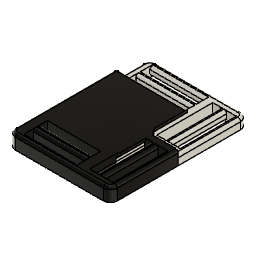
Bickle v11 (Autodesk Fusion 360 design; units mm, degrees)
Autodesk Fusion 360 part; units mm, degrees
sketch "Sketch1" plane through (0, 0, 0) normal (0, 0, 1) x (1, 0, 0)
  line L0 (0, 0) -> (50.5, 0)
  line L1 (0, 0) -> (5, 0)
  line L2 (5, 0) -> (5, -5) construction
  line L3 (0, 0) -> (0, -5)
  line L4 (50.5, 0) -> (50.5, -5)
  line L5 (50.5, -5) -> (45.5, -5)
  line L6 (45.5, -5) -> (45.5, 0) construction
  line L7 (45.5, -5) -> (0, -5)
  line L8 (0, -5) -> (0, -10)
  line L9 (0, -10) -> (50.5, -10)
  line L10 (50.5, -5) -> (50.5, -10)
  line L11 (0, 0) -> (0, 5)
  line L12 (0, 5) -> (51, 5)
  line L13 (50.5, 0) -> (50.5, 5)
  line L14 (0, -10) -> (0, -65)
  line L15 (50.5, -10) -> (50.5, -65)
  line L16 (50.5, -65) -> (0, -65)
  line L17 (45.5, 5) -> (45.5, -10)
  line L18 (5, -5) -> (5, -10)
  line L19 (5, 0) -> (5, 5)
  line L20 (50.5, 5) -> (50.5, 10)
  line L21 (50.5, 10) -> (0, 10)
  line L22 (0, 10) -> (0, 5)
  dimension "d1" = 50.5
  dimension "d2" = 5
  dimension "d3" = 5
  dimension "d4" = 5
  dimension "d5" = 5
  dimension "d6" = 5
  dimension "d7" = 5
  dimension "d8" = 5
  dimension "d11" = 55
  dimension "d12" = 55
  dimension "d13" = 5
  constraint coincident L0.start L1.start
  constraint horizontal L0
  constraint parallel L0 L1
  constraint perpendicular L0 L2
  constraint perpendicular L1 L3
  constraint perpendicular L0 L4
  constraint perpendicular L4 L5
  constraint coincident L0 L6.end
  constraint perpendicular L0 L6
  constraint perpendicular L7 L8
  constraint perpendicular L8 L9
  constraint coincident L9 L10.end
  constraint perpendicular L9 L10
  constraint perpendicular L1 L11
  constraint perpendicular L11 L12
  constraint coincident L12 L13.end
  constraint perpendicular L12 L13
  constraint perpendicular L9 L14
  constraint perpendicular L9 L15
  constraint coincident L12 L17.start
  constraint coincident L9 L17.end
  constraint perpendicular L9 L17
  constraint coincident L9 L18.end
  constraint perpendicular L9 L18
  constraint coincident L12 L19.end
  constraint perpendicular L12 L19
  constraint perpendicular L12 L20
  constraint perpendicular L20 L21
  constraint coincident L12 L11.end
  constraint perpendicular L12 L22
  measures "d1" distance of L0.start L0.end
  measures "d2" distance of L0.start L1.end
  measures "d3" distance of L1.end L2.end
  measures "d4" distance of L0.start L3.end
  measures "d5" distance of L0.end L4.end
  measures "d6" distance of L4.end L5.end
  measures "d7" distance of L3.end L8.end
  measures "d8" distance of L0.start L11.end
  measures "d11" distance of L8.end L14.end
  measures "d12" distance of L9.end L15.end
  measures "d13" distance of L13.end L20.end
extrude "Extrude2" add sketch "Sketch1" along normal blind 7 contours L0 L1 L11 L12 L19 | L0 L1 L3 L7 L17 | L7 L8 L9 L18 | L12 L20 L21 L22 | L0 L12 L13 L17 | L0 L4 L5 L17 | L9 L14 L15 L16 | L5 L9 L10 L17 makes body 1
fillet "Fillet1" radius 2 4 edges at (25.25, 0, 0) (25.25, -5, 0) (25.25, -5, 7) (25.25, 0, 7) on bodies 1
sketch "Sketch2" plane through (0, 0, 0) normal (0, 0, -1) x (1, 0, 0)
  line L0 (45.5, 10) -> (45.5, 3)
  line L1 (45.5, 3) -> (5, 3)
  line L2 (5, 3) -> (5, 10)
  line L3 (5, 10) -> (45.5, 10)
  line L4 (5, -5) -> (5, 2)
  line L5 (5, 2) -> (45.5, 2)
  line L6 (45.5, 2) -> (45.5, -5)
  line L7 (45.5, -5) -> (5, -5)
  line L8 (50.5, -10) -> (50.5, 65)
  line L9 (50.5, 65) -> (0, 65)
  line L10 (0, 65) -> (0, -10)
  line L11 (0, -10) -> (50.5, -10)
  line L12 (50.5, -10) -> (70.5, -10)
  line L13 (70.5, -10) -> (70.5, 40.5)
  line L14 (70.5, 40.5) -> (50.5, 65)
  line L15 (70.5, 40.5) -> (50.5, 40.5)
  line L16 (50.5, -10) -> (55.5, -10)
  line L17 (55.5, -10) -> (60.5, -10)
  line L18 (60.5, -10) -> (65.5, -10)
  line L19 (65.5, -10) -> (65.5, 40.5)
  line L20 (60.5, -10) -> (60.5, 40.5)
  line L21 (55.5, -10) -> (55.5, 40.5)
  line L22 (50.5, -10) -> (50.5, -5)
  line L23 (50.5, -5) -> (70.5, -5)
  line L24 (70.5, 40.5) -> (70.5, 35.5)
  line L25 (70.5, 35.5) -> (50.5, 35.5)
  dimension "d18" = 20
  dimension "d19" = 50.5
  dimension "d20" = 5
  dimension "d21" = 5
  dimension "d22" = 5
  dimension "d23" = 5
  constraint coincident L8.start L11.end
  constraint perpendicular L8 L12
  constraint perpendicular L12 L13
  constraint coincident L8.end L9.start
  constraint coincident L8 L15.end
  constraint perpendicular L8 L15
  constraint perpendicular L8 L16
  constraint parallel L12 L17
  constraint coincident L12 L18.end
  constraint coincident L15 L19.end
  constraint perpendicular L15 L19
  constraint midpoint L15 L20.end
  constraint coincident L15 L21.end
  constraint perpendicular L15 L21
  constraint coincident L8 L22.end
  constraint perpendicular L16 L22
  constraint coincident L13 L23.end
  constraint perpendicular L13 L23
  constraint perpendicular L15 L24
  constraint coincident L8 L25.end
  constraint perpendicular L8 L25
  measures "d18" distance of L8.start L12.end
  measures "d19" distance of L12.end L13.end
  measures "d20" distance of L8.start L16.end
  measures "d21" distance of L16.end L17.end
  measures "d22" distance of L17.end L18.end
  measures "d23" distance of L13.end L24.end
extrude "Extrude3" add sketch "Sketch2" against normal up to surface (7 mm away) contours L8 L12 L16 L21 L22 L23 | L12 L17 L20 L21 L23 | L8 L15 L21 L25 | L20 L21 L23 L25 | L12 L18 L19 L20 L23 | L15 L20 L21 L25 | L12 L13 L19 L23 | L15 L19 L20 L25 | L13 L19 L23 L25 | L13 L15 L19 L24 L25 bodies 1
fillet "Fillet2" radius 2 4 edges at (60.5, -15.25, 7) (60.5, -15.25, 0) (55.5, -15.25, 7) (55.5, -15.25, 0) on bodies 1
sketch "Sketch3" plane through (0, 0, 7) normal (0, 0, 1) x (-1, 0, 0)
  line L0 (-70.5, -10) -> (0, -10)
  line L1 (0, -10) -> (0, 65)
  line L2 (0, 65) -> (-50.5, 65)
  line L3 (-70.5, 40.5) -> (-70.5, -10)
  line L4 (-65.5, 35.5) -> (-58.5, 35.5)
  line L5 (-58.5, 35.5) -> (-58.5, -5)
  line L6 (-58.5, -5) -> (-65.5, -5)
  line L7 (-65.5, -5) -> (-65.5, 35.5)
  line L8 (-5, 2) -> (-5, -5)
  line L9 (-5, -5) -> (-45.5, -5)
  line L10 (-45.5, -5) -> (-45.5, 2)
  line L11 (-45.5, 2) -> (-5, 2)
  line L12 (-45.5, 3) -> (-45.5, 10)
  line L13 (-45.5, 10) -> (-5, 10)
  line L14 (-5, 10) -> (-5, 3)
  line L15 (-5, 3) -> (-45.5, 3)
  line L16 (-50.5, -5) -> (-57.5, -5)
  line L17 (-57.5, -5) -> (-57.5, 35.5)
  line L18 (-57.5, 35.5) -> (-50.5, 35.5)
  line L19 (-50.5, 65) -> (-50.5, 40.5)
  line L20 (-25.25, 10) -> (-25.25, 65) construction
  line L21 (-45.5, 10) -> (-51, 10) construction
  line L22 (-50.5, 65) -> (-50.5, 10) construction
  circle A0 centre (-25.25, 37.5) radius 12.25
  line L23 (-70.5, 40.5) -> (0, 40.5) construction
  line L24 (-25.25, 49.75) -> (-25.25, 47.75) construction
  line L25 (-25.25, 47.75) -> (-18.5418, 47.75)
  line L26 (-25.25, 37.5) -> (-13, 37.5) construction
  line L27 (-18.5418, 47.75) -> (-13, 37.5)
  line L28 (-25.25, 37.5) -> (-39, 37.5) construction
  line L29 (-25.25, 47.75) -> (-31.9582, 47.75)
  line L30 (-31.9582, 47.75) -> (-37.5, 37.5)
  line L31 (-21.8959, 47.75) -> (-21.8959, 65)
  line L32 (-28.6041, 47.75) -> (-28.6041, 65)
  line L33 (-21.8959, 47.75) -> (-21.8959, 52.75)
  line L34 (-21.8959, 52.75) -> (-28.6041, 52.75)
  line L35 (-50.5, 40.5) -> (-70.5, 40.5)
  line L36 (-50.5, 35.5) -> (-50.5, -5)
  dimension "d28" = 2
  dimension "d31" = 5
  dimension "d38" = 24.5
  constraint midpoint L13 L20.start
  constraint midpoint L2 L20.end
  constraint coincident L12.end L13.start
  constraint perpendicular L19 L21
  constraint coincident L2.end L19.start
  constraint coincident L21 L22.end
  constraint coincident L19 L22.end
  constraint midpoint L20 A0.centre
  constraint coincident L3.start L23.start
  constraint coincident L1 L23.end
  constraint perpendicular L1 L23
  constraint coincident A0 L24.start
  constraint coincident L20 L24.start
  constraint parallel L20 L24
  constraint coincident A0 L25.end
  constraint perpendicular L24 L25
  constraint coincident A0.centre L26.start
  constraint coincident A0 L26.end
  constraint perpendicular L20 L26
  constraint perpendicular L20 L28
  constraint perpendicular L24 L29
  constraint coincident A0 L29.end
  constraint coincident L29 L30.start
  constraint coincident A0 L30.end
  constraint coincident L28 L30.end
  constraint midpoint L25 L31.start
  constraint coincident L2 L31.end
  constraint perpendicular L2 L31
  constraint midpoint L29 L32.start
  constraint coincident L2 L32.end
  constraint perpendicular L2 L32
  constraint perpendicular L25 L33
  constraint coincident L32 L34.end
  constraint perpendicular L32 L34
  measures "d28" distance of L24.start L24.end
  measures "d31" distance of L31.start L33.end
  measures "d38" diameter of A0
extrude "Extrude4" cut sketch "Sketch3" against normal blind 5 contours A0 L31 L32 L33 L34 | A0 L25 L29 L31 L32 L33 | A0 L25 L27 L29 L30 bodies 1
sketch "Sketch4" plane through (0, 0, 2) normal (0, 0, 1) x (-1, 0, 0)
  line L0 (-21.8959, 47.75) -> (-21.8959, 52.75)
  line L1 (-21.8959, 52.75) -> (-28.6041, 52.75)
  line L2 (-28.6041, 52.75) -> (-28.6041, 47.75)
  line L3 (-28.6041, 47.75) -> (-31.9582, 47.75)
  line L4 (-31.9582, 47.75) -> (-37.5, 37.5)
  arc A0 (-37.5, 37.5) -> (-13, 37.5) centre (-25.25, 37.5) ccw
  line L5 (-13, 37.5) -> (-18.5418, 47.75)
  line L6 (-18.5418, 47.75) -> (-21.8959, 47.75)
  circle A1 centre (-25.25, 37.5) radius 12.25
  line L7 (-25.25, 37.5) -> (-25.25, 52.75)
  line L8 (-25.25, 37.5) -> (-25.25, 47.5)
  circle A2 centre (-25.25, 47.5) radius 12.25
  line L9 (-13, 37.5) -> (-13, 47.5)
  line L10 (-37.5, 37.5) -> (-37.5, 47.5)
  dimension "d32" = 10
  dimension "d33" = 24.5
  dimension "d34" = 24.5
  constraint concentric A0 A1
  constraint coincident A0.centre A1.centre
  constraint midpoint L1 L7.end
  constraint parallel L7 L8
  constraint coincident L8.end A2.centre
  constraint coincident A0.end L5.start
  constraint coincident A2 L9.end
  constraint tangent A2 L9
  constraint coincident L4.end A0.start
  constraint coincident A2 L10.end
  constraint tangent A2 L10
  measures "d32" distance of A0.centre L8.end
  measures "d33" diameter of A1
  measures "d34" diameter of A2
extrude "Extrude5" cut sketch "Sketch4" along normal blind 3 contours L0 L2 L3 L4 L5 L6 A1 A2 | L0 L6 A1 | L0 L1 A1 L7 | L0 L1 L2 A1 A2 | L5 A1 A2 | L1 L2 A1 L7 | L5 A1 A2 | A1 A2 L9 | L2 L3 A1 | L4 A1 A2 | L4 A1 A2 | A1 A2 L10 bodies 1
sketch "Sketch1 (2)" plane through (0, 0, 2) normal (0, 0, 1) x (-1, 0, 0) in component "Topo"
  arc A0 (-37.5, 37.5) -> (-13, 37.5) centre (-25.25, 37.5) ccw
  line L0 (-13, 37.5) -> (-13, 47.5)
  arc A1 (-13, 47.5) -> (-37.5, 47.5) centre (-25.25, 47.5) ccw
  line L1 (-37.5, 47.5) -> (-37.5, 37.5)
  circle A2 centre (-25.25, 37.5) radius 10.7848
  point P0 (-28.6041, 47.75)
  constraint concentric A0 A2
  constraint coincident P0 A2
extrude "Extrude1" add sketch "Sketch1 (2)" along normal blind 2 separate body contours A2 makes body 2 in component "Topo"
fillet "Fillet3" radius 1 2 edges at (21.8959, -47.75, 6) (28.6041, -47.75, 6) on bodies 1
sketch "Sketch2 (2)" plane through (0, 0, 4) normal (0, 0, 1) x (-1, 0, 0) in component "Topo"
  circle A0 centre (-25.25, 37.5) radius 10.7848
  line L0 (-28.6041, 41.75) -> (-21.8959, 41.75)
  line L1 (-21.8959, 41.75) -> (-21.8959, 37.75)
  line L2 (-20.8959, 36.75) -> (-18.5418, 36.75)
  line L3 (-18.5418, 36.75) -> (-13, 26.5)
  arc A1 (-37.5, 26.5) -> (-13, 26.5) centre (-25.25, 26.5) ccw
  line L4 (-37.5, 26.5) -> (-31.9582, 36.75)
  line L5 (-31.9582, 36.75) -> (-29.6041, 36.75)
  line L6 (-28.6041, 37.75) -> (-28.6041, 41.75)
  line L7 (-70.5, -21) -> (0, -21)
  line L8 (0, -21) -> (0, 54)
  line L9 (0, 54) -> (-50.5, 54)
  line L10 (-70.5, 29.5) -> (-70.5, -21)
  line L11 (-65.5, 24.5) -> (-58.5, 24.5)
  line L12 (-58.5, 24.5) -> (-58.5, -16)
  line L13 (-58.5, -16) -> (-65.5, -16)
  line L14 (-65.5, -16) -> (-65.5, 24.5)
  line L15 (-5, -9) -> (-5, -16)
  line L16 (-5, -16) -> (-45.5, -16)
  line L17 (-45.5, -16) -> (-45.5, -9)
  line L18 (-45.5, -9) -> (-5, -9)
  line L19 (-45.5, -8) -> (-45.5, -1)
  line L20 (-45.5, -1) -> (-5, -1)
  line L21 (-5, -1) -> (-5, -8)
  line L22 (-5, -8) -> (-45.5, -8)
  line L23 (-50.5, -16) -> (-57.5, -16)
  line L24 (-57.5, -16) -> (-57.5, 24.5)
  line L25 (-57.5, 24.5) -> (-50.5, 24.5)
  line L26 (-50.5, 54) -> (-50.5, 29.5)
  arc A2 (-29.6041, 36.75) -> (-28.6041, 37.75) centre (-29.6041, 37.75) ccw
  arc A3 (-21.8959, 37.75) -> (-20.8959, 36.75) centre (-20.8959, 37.75) ccw
  line L27 (-22.3959, 41.25) -> (-22.3959, 37.75)
  arc A4 (-22.3959, 37.75) -> (-20.8959, 36.25) centre (-20.8959, 37.75) ccw
  line L28 (-20.8959, 36.25) -> (-18.8399, 36.25)
  line L29 (-18.8399, 36.25) -> (-13.5007, 26.3747)
  arc A5 (-36.9993, 26.3747) -> (-13.5007, 26.3747) centre (-25.25, 26.5) ccw
  line L30 (-36.9993, 26.3747) -> (-31.6601, 36.25)
  line L31 (-31.6601, 36.25) -> (-29.6041, 36.25)
  arc A6 (-29.6041, 36.25) -> (-28.1041, 37.75) centre (-29.6041, 37.75) ccw
  line L32 (-28.1041, 37.75) -> (-28.1041, 41.25)
  line L33 (-28.1041, 41.25) -> (-22.3959, 41.25)
  line L34 (-50.5, 29.5) -> (-70.5, 29.5)
  line L35 (-50.5, 24.5) -> (-50.5, -16)
  dimension "d43" = 0.5
extrude "Extrude2'" add sketch "Sketch2 (2)" along normal up to surface (3 mm away) contours A0 L27 A4 L28 L29 L30 L31 A6 L32 L33 bodies 2 in component "Topo"
extrude "Extrude3'" add 1 faces at (25.25, -33.316, 7) along direction (0, 0, 1) blind 1 on bodies 2 bodies 2 in component "Topo"
move_body "Move1" bodies 2 to x (1, 0, 0) y (0, 1, 0) z (0, 0, 1) at (0, 11, 0) in component "Topo"
sketch "Sketch4 (2)" plane through (0, 0, 8) normal (0, 0, 1) x (-1, 0, 0) in component "Topo"
  line L0 (-31.6601, 25.25) -> (-34.2209, 20.5137)
  arc A0 (-34.2209, 20.5137) -> (-16.2791, 20.5137) centre (-25.25, 26.5) ccw
  line L1 (-16.2791, 20.5137) -> (-18.8399, 25.25)
  line L2 (-18.8399, 25.25) -> (-20.8959, 25.25)
  arc A1 (-22.3959, 26.75) -> (-20.8959, 25.25) centre (-20.8959, 26.75) ccw
  line L3 (-22.3959, 26.75) -> (-22.3959, 30.25)
  line L4 (-22.3959, 30.25) -> (-28.1041, 30.25)
  line L5 (-28.1041, 30.25) -> (-28.1041, 26.75)
  arc A2 (-29.6041, 25.25) -> (-28.1041, 26.75) centre (-29.6041, 26.75) ccw
  line L6 (-29.6041, 25.25) -> (-31.6601, 25.25)
  arc A3 (-29.6041, 36.75) -> (-28.6041, 37.75) centre (-29.6041, 37.75) ccw
  line L7 (-28.6041, 37.75) -> (-28.6041, 41.75)
  line L8 (-28.6041, 41.75) -> (-21.8959, 41.75)
  line L9 (-21.8959, 41.75) -> (-21.8959, 37.75)
  arc A4 (-21.8959, 37.75) -> (-20.8959, 36.75) centre (-20.8959, 37.75) ccw
  line L10 (-20.8959, 36.75) -> (-18.5418, 36.75)
  line L11 (-18.5418, 36.75) -> (-13, 26.5)
  arc A5 (-37.5, 26.5) -> (-13, 26.5) centre (-25.25, 26.5) ccw
  line L12 (-37.5, 26.5) -> (-31.9582, 36.75)
  line L13 (-31.9582, 36.75) -> (-29.6041, 36.75)
  line L14 (-70.5, -21) -> (0, -21)
  line L15 (0, -21) -> (0, 54)
  line L16 (0, 54) -> (-50.5, 54)
  line L17 (-70.5, 29.5) -> (-70.5, -21)
  line L18 (-65.5, 24.5) -> (-58.5, 24.5)
  line L19 (-58.5, 24.5) -> (-58.5, -16)
  line L20 (-58.5, -16) -> (-65.5, -16)
  line L21 (-65.5, -16) -> (-65.5, 24.5)
  line L22 (-5, -9) -> (-5, -16)
  line L23 (-5, -16) -> (-45.5, -16)
  line L24 (-45.5, -16) -> (-45.5, -9)
  line L25 (-45.5, -9) -> (-5, -9)
  line L26 (-45.5, -8) -> (-45.5, -1)
  line L27 (-45.5, -1) -> (-5, -1)
  line L28 (-5, -1) -> (-5, -8)
  line L29 (-5, -8) -> (-45.5, -8)
  line L30 (-50.5, -16) -> (-57.5, -16)
  line L31 (-57.5, -16) -> (-57.5, 24.5)
  line L32 (-57.5, 24.5) -> (-50.5, 24.5)
  line L33 (-50.5, 54) -> (-50.5, 29.5)
  line L34 (0, -1) -> (0, 1)
  line L35 (-50.5, 24.5) -> (-48.5, 24.5)
  line L36 (-48.5, 24.5) -> (-48.5, 54)
  line L37 (-48.5, 24.5) -> (-48.5, -2)
  line L38 (0, 1) -> (-48.5, 1)
  line L39 (-48.5, 54) -> (-48.5, 59)
  line L40 (0, 54) -> (0, 59)
  line L41 (0, 59) -> (-48.5, 59)
  line L42 (0, 59) -> (0, 64)
  line L43 (0, 64) -> (0, 69)
  line L44 (0, 69) -> (0, 74)
  line L45 (0, 64) -> (-49, 64)
  line L46 (0, 69) -> (-51, 69)
  line L47 (0, 74) -> (-52, 74)
  line L48 (-48.5, 59) -> (-48.5, 74)
  line L49 (0, 54) -> (-5, 54)
  line L50 (-5, 54) -> (-5, 74)
  line L51 (-48.5, 54) -> (-43.5, 54)
  line L52 (-43.5, 54) -> (-43.5, 74)
  line L53 (-70.5, 29.5) -> (-48.5, 29.5)
  line L54 (-50.5, 29.5) -> (-70.5, 29.5)
  line L55 (-50.5, 24.5) -> (-50.5, -16)
  line L56 (-31.6601, 25.25) -> (-34.2209, 20.5137)
  arc A6 (-34.2209, 20.5137) -> (-16.2791, 20.5137) centre (-25.25, 26.5) ccw
  line L57 (-16.2791, 20.5137) -> (-18.8399, 25.25)
  line L58 (-18.8399, 25.25) -> (-20.8959, 25.25)
  arc A7 (-22.3959, 26.75) -> (-20.8959, 25.25) centre (-20.8959, 26.75) ccw
  line L59 (-22.3959, 26.75) -> (-22.3959, 30.25)
  line L60 (-22.3959, 30.25) -> (-28.1041, 30.25)
  line L61 (-28.1041, 30.25) -> (-28.1041, 26.75)
  arc A8 (-29.6041, 25.25) -> (-28.1041, 26.75) centre (-29.6041, 26.75) ccw
  line L62 (-29.6041, 25.25) -> (-31.6601, 25.25)
  line L63 (0, 79) -> (-53, 79)
  line L64 (-48.5, 74) -> (-48.5, 79)
  line L65 (0, 79) -> (0, 74)
  line L66 (-43.5, 74) -> (-43.5, 79)
  line L67 (-5, 74) -> (-5, 79)
  dimension "d48" = 2
  dimension "d49" = 2
  dimension "d52" = 5
  dimension "d53" = 5
  dimension "d54" = 5
  dimension "d55" = 5
  dimension "d56" = 5
  dimension "d57" = 5
  dimension "d58" = 5
  constraint coincident L15 L34.start
  constraint perpendicular L27 L34
  constraint coincident L16.end L32.end
  constraint perpendicular L33 L35
  constraint coincident L16 L36.end
  constraint perpendicular L16 L36
  constraint perpendicular L35 L37
  constraint coincident L37 L38.end
  constraint perpendicular L37 L38
  constraint perpendicular L16 L39
  constraint coincident L15.end L16.start
  constraint perpendicular L16 L40
  constraint perpendicular L41 L42
  constraint parallel L42 L43
  constraint parallel L43 L44
  constraint perpendicular L42 L45
  constraint perpendicular L44 L46
  constraint perpendicular L44 L47
  constraint coincident L47 L48.end
  constraint perpendicular L47 L48
  constraint perpendicular L15 L49
  constraint coincident L47 L50.end
  constraint perpendicular L47 L50
  constraint perpendicular L39 L51
  constraint coincident L47 L52.end
  constraint perpendicular L47 L52
  constraint coincident L17.start L53.start
  constraint coincident L36 L53.end
  constraint perpendicular L36 L53
  measures "d48" distance of L34.start L34.end
  measures "d49" distance of L32.end L35.end
  measures "d52" distance of L36.end L39.end
  measures "d53" distance of L15.end L40.end
  measures "d54" distance of L40.end L42.end
  measures "d55" distance of L42.end L43.end
  measures "d56" distance of L43.end L44.end
  measures "d57" distance of L15.end L49.end
  measures "d58" distance of L36.end L51.end
extrude "Extrude5'" add sketch "Sketch4 (2)" along normal blind 2 contours L0 A0 L1 L2 A1 L3 L4 L5 A2 L6 L56 A6 L57 L58 A7 L59 L60 L61 A8 L62 | A3 L7 L8 L9 A4 L10 L11 A5 L12 L13 | L15 L16 L36 L37 L38 L49 L51 | L16 L40 L41 L49 L50 | L16 L39 L41 L51 L52 | L16 L41 L50 L52 | L41 L42 L45 L50 | L41 L45 L48 L52 | L43 L45 L46 L50 | L45 L46 L48 L52 | L45 L46 L50 L52 | L44 L46 L47 L50 | L46 L47 L48 L52 | L47 L63 L65 L67 | L47 L63 L64 L66 | L47 L63 L66 L67 bodies 2 in component "Topo"
extrude "Extrude4'" add sketch "Sketch4 (2)" along normal blind 2 contours L0 A0 L1 L2 A1 L3 L4 L5 A2 L6 L56 A6 L57 L58 A7 L59 L60 L61 A8 L62 | A3 L7 L8 L9 A4 L10 L11 A5 L12 L13 | L15 L16 L36 L37 L38 L49 L51 bodies 2 in component "Topo"
extrude "Extrude6" add sketch "Sketch4 (2)" along normal blind 2 contours L16 L33 L36 L53 bodies 2 in component "Topo"
sketch "Sketch5" plane through (0, 0, 10) normal (0, 0, 1) x (-1, 0, 0) in component "Topo"
  line L0 (-43.5, 59) -> (-43.5, 64)
  line L1 (-5, 59) -> (-43.5, 59)
  line L2 (-5, 64) -> (-5, 59)
  line L3 (-48.5, 79) -> (-48.5, 54)
  line L4 (-48.5, 54) -> (-50.5, 54)
  line L5 (-50.5, 54) -> (-50.5, 29.5)
  line L6 (-50.5, 29.5) -> (-48.5, 29.5)
  line L7 (-48.5, 29.5) -> (-48.5, 1)
  line L8 (-48.5, 1) -> (0, 1)
  line L9 (0, 1) -> (0, 79)
  line L10 (-43.5, 74) -> (-5, 74)
  line L11 (-5, 69) -> (-43.5, 69)
  line L12 (-5, 74) -> (-5, 69)
  line L13 (-43.5, 64) -> (-5, 64)
  line L14 (-43.5, 69) -> (-43.5, 74)
  line L15 (-50.5, 54) -> (-70.5, 29.5)
  line L16 (-70.5, 29.5) -> (-50.5, 29.5)
  line L17 (-50.5, 29.5) -> (-50.5, 54)
  line L18 (-50.5, 29.5) -> (-51.5, 29.5)
  line L19 (-51.5, 29.5) -> (-51.5, 52.775)
  line L20 (0, 79) -> (-48.5, 79)
  point P0 (-50.5, 29.5)
  dimension "d65" = 1
  constraint coincident P0 L5.end
  constraint perpendicular L17 L18
  constraint coincident L15 L19.end
  constraint perpendicular L18 L19
  measures "d65" distance of P0 L18.end
extrude "Extrude7" add sketch "Sketch5" against normal blind 2 contours L5 L15 L16 L17 L18 L19 bodies 2 in component "Topo"
sketch "Sketch6" plane through (0, 0, 10) normal (0, 0, 1) x (-1, 0, 0) in component "Topo"
  line L0 (-43.5, 59) -> (-43.5, 64)
  line L1 (-5, 59) -> (-43.5, 59)
  line L2 (-5, 64) -> (-5, 59)
  line L3 (-48.5, 79) -> (-48.5, 54)
  line L4 (-48.5, 54) -> (-50.5, 54)
  line L5 (-50.5, 54) -> (-51.5, 52.775)
  line L6 (-51.5, 52.775) -> (-51.5, 29.5)
  line L7 (-51.5, 29.5) -> (-48.5, 29.5)
  line L8 (-48.5, 29.5) -> (-48.5, 1)
  line L9 (-48.5, 1) -> (0, 1)
  line L10 (0, 1) -> (0, 79)
  line L11 (-43.5, 74) -> (-5, 74)
  line L12 (-5, 69) -> (-43.5, 69)
  line L13 (-5, 74) -> (-5, 69)
  line L14 (-43.5, 64) -> (-5, 64)
  line L15 (-43.5, 69) -> (-43.5, 74)
  line L16 (-51.5, 29.5) -> (-51.5, 52.775)
  line L17 (-51.5, 52.775) -> (-70.5, 29.5)
  line L18 (-70.5, 29.5) -> (-51.5, 29.5)
  line L19 (-48.5, 79) -> (-79, 79)
  line L20 (-70.5, 29.5) -> (-70.5, 79)
  arc A0 (-29.6041, 36.75) -> (-28.6041, 37.75) centre (-29.6041, 37.75) ccw
  line L21 (-28.6041, 37.75) -> (-28.6041, 41.75)
  line L22 (-28.6041, 41.75) -> (-21.8959, 41.75)
  line L23 (-21.8959, 41.75) -> (-21.8959, 37.75)
  arc A1 (-21.8959, 37.75) -> (-20.8959, 36.75) centre (-20.8959, 37.75) ccw
  line L24 (-20.8959, 36.75) -> (-18.5418, 36.75)
  line L25 (-18.5418, 36.75) -> (-13, 26.5)
  arc A2 (-37.5, 26.5) -> (-13, 26.5) centre (-25.25, 26.5) ccw
  line L26 (-37.5, 26.5) -> (-31.9582, 36.75)
  line L27 (-31.9582, 36.75) -> (-29.6041, 36.75)
  line L28 (-70.5, -21) -> (0, -21)
  line L29 (0, -21) -> (0, 54)
  line L30 (0, 54) -> (-50.5, 54)
  line L31 (-50.5, 54) -> (-50.5, 29.5)
  line L32 (-50.5, 29.5) -> (-70.5, 29.5)
  line L33 (-70.5, 29.5) -> (-70.5, -21)
  line L34 (-65.5, 24.5) -> (-58.5, 24.5)
  line L35 (-58.5, 24.5) -> (-58.5, -16)
  line L36 (-58.5, -16) -> (-65.5, -16)
  line L37 (-65.5, -16) -> (-65.5, 24.5)
  line L38 (-5, -9) -> (-5, -16)
  line L39 (-5, -16) -> (-45.5, -16)
  line L40 (-45.5, -16) -> (-45.5, -9)
  line L41 (-45.5, -9) -> (-5, -9)
  line L42 (-45.5, -8) -> (-45.5, -1)
  line L43 (-45.5, -1) -> (-5, -1)
  line L44 (-5, -1) -> (-5, -8)
  line L45 (-5, -8) -> (-45.5, -8)
  line L46 (-50.5, -16) -> (-57.5, -16)
  line L47 (-57.5, -16) -> (-57.5, 24.5)
  line L48 (-57.5, 24.5) -> (-50.5, 24.5)
  line L49 (-50.5, 24.5) -> (-50.5, -16)
  line L50 (-65.5, 24.5) -> (-65.5, 79)
  line L51 (-50.5, 24.5) -> (-50.5, 79)
  line L52 (-50.5, 79) -> (-55.5, 79)
  line L53 (-65.5, 79) -> (-60.5, 79)
  line L54 (-60.5, 79) -> (-60.5, 29.5)
  line L55 (-55.5, 79) -> (-55.5, 24.5)
  line L56 (-50.5, 29.5) -> (-70.5, 29.5)
  line L57 (-70.5, 29.5) -> (-70.5, 34.5)
  line L58 (0, 79) -> (-48.5, 79)
  line L59 (-70.5, 79) -> (-70.5, 74)
  line L60 (-70.5, 29.5) -> (-70.5, 34.5)
  line L61 (-70.5, 34.5) -> (-50, 34.5)
  line L62 (-70.5, 74) -> (-49, 74)
  dimension "d71" = 5
  dimension "d74" = 5
  dimension "d75" = 5
  constraint coincident L3.start L19.start
  constraint perpendicular L3 L19
  constraint coincident L17.end L18.start
  constraint coincident L19 L20.end
  constraint perpendicular L19 L20
  constraint coincident L34.start L37.end
  constraint coincident L19 L50.end
  constraint perpendicular L19 L50
  constraint coincident L48.end L49.start
  constraint coincident L19 L51.end
  constraint perpendicular L19 L51
  constraint perpendicular L51 L52
  constraint perpendicular L50 L53
  constraint midpoint L32 L54.end
  constraint coincident L48 L55.end
  constraint perpendicular L48 L55
  constraint coincident L31.end L32.start
  constraint perpendicular L56 L57
  constraint perpendicular L19 L59
  constraint parallel L20 L60
  constraint perpendicular L51 L61
  constraint perpendicular L51 L62
  measures "d71" distance of L50.end L53.end
  measures "d74" distance of L20.end L59.end
  measures "d75" distance of L17.end L57.end
extrude "Extrude9" add sketch "Sketch6" against normal blind 10 contours L3 L4 L19 L30 L51 | L19 L51 L52 L55 L62 | L19 L54 L55 L62 | L19 L50 L53 L54 L62 | L17 L54 L55 L62 | L6 L16 L18 L32 L55 L56 L61 | L17 L54 L55 L61 | L19 L20 L50 L59 L62 | L18 L32 L54 L55 L56 L61 | L17 L20 L50 L61 L62 | L18 L32 L50 L54 L56 L61 | L17 L50 L61 | L17 L20 L57 L60 L61 | L17 L18 L32 L50 L56 L61 bodies 2 in component "Topo"
fillet "Fillet1'" radius 2 4 edges at (55.5, -54.25, 10) (60.5, -54.25, 10) (55.5, -54.25, 0) (60.5, -54.25, 0) on bodies 2 in component "Topo"
extrude "Extrude10" add sketch "Sketch4 (2)" against normal blind 8 contours L16 L40 L41 L49 L50 | L16 L39 L41 L51 L52 | L16 L41 L50 L52 | L41 L42 L45 L50 | L41 L45 L48 L52 | L43 L45 L46 L50 | L45 L46 L48 L52 | L45 L46 L50 L52 | L44 L46 L47 L50 | L46 L47 L48 L52 | L47 L63 L65 L67 | L47 L63 L64 L66 | L47 L63 L66 L67 bodies 2 in component "Topo"
fillet "Fillet2'" radius 2 4 edges at (24.25, -69, 10) (24.25, -64, 10) (24.25, -69, 0) (24.25, -64, 0) on bodies 2 in component "Topo"
chamfer "Chamfer2" distance 2 angle 45 2 edges at (65.5, -15.25, 7) (25.25, 5, 7) on bodies 1
chamfer "Chamfer1" distance 2 angle 45 2 edges at (65.5, -54.25, 10) (24.25, -74, 10) on bodies 2 in component "Topo"
chamfer "Chamfer3" distance 2 angle 45 2 edges at (65.5, -15.25, 0) (25.25, 5, 0) on bodies 1
chamfer "Chamfer2'" distance 2 angle 45 2 edges at (24.25, -74, 0) (65.5, -54.25, 0) on bodies 2 in component "Topo"
fillet "Fillet4" radius 1 1 edges at (25.25, -37.2848, 4) on bodies 2 in component "Topo"
copy_body "Body->Comp1" bodies 1 removing the originals makes body 3 in component "Trinco"
fillet "Fillet5" radius 5 1 edges at (50.5, -64, 0) on bodies 2 in component "Topo"
sketch "Sketch5 (2)" plane through (0, 0, 0) normal (-1, 0, 0) x (0, -1, 0)
  line L0 (23, 8) -> (76, 8)
  line L1 (76, 8) -> (76, 0)
  line L2 (76, 0) -> (101, 0)
  line L3 (101, 0) -> (101, 10)
  line L4 (101, 10) -> (23, 10)
  line L5 (23, 10) -> (23, 8)
  line L6 (23, 10) -> (23, -2)
  line L7 (23, -2) -> (23, 0)
  line L8 (101, 0) -> (23, 0)
  constraint coincident L4.end L5.start
  constraint perpendicular L0 L6
  constraint coincident L6 L7.end
  constraint coincident L2.end L3.start
  constraint perpendicular L7 L8
extrude "Extrude11" add sketch "Sketch5 (2)" along normal blind 1 contours L0 L1 L2 L3 L4 L5 L6 L8 sketch seen with x (1, 0, 0) y (0, 1, 0) z (0, 0, 1) at (0, 22, 0) bodies 2 in component "Topo"
sketch "Sketch6 (2)" plane through (-1, 0, 0) normal (-1, 0, 0) x (0, -1, 0)
  line L0 (101, 10) -> (23, 10)
  line L1 (23, 10) -> (23, 8)
  line L2 (23, 8) -> (76, 8)
  line L3 (76, 8) -> (76, 0)
  line L4 (76, 0) -> (101, 0)
  line L5 (101, 0) -> (101, 10)
  line L6 (23, 10) -> (23, -2)
  line L7 (101, 0) -> (23, 0)
  constraint coincident L0.end L1.start
  constraint perpendicular L0 L6
  constraint coincident L4.end L5.start
  constraint coincident L6 L7.end
  constraint perpendicular L6 L7
extrude "Extrude12" add sketch "Sketch6 (2)" along normal blind 2 sketch seen with x (1, 0, 0) y (0, 1, 0) z (0, 0, 1) at (0, 22, 0) bodies 2 in component "Topo"
fillet "Fillet1''" radius 5 2 edges at (0, 10, 3.5) (70.5, 10, 3.5) on bodies 3 in component "Trinco"
fillet "Fillet6" radius 5 2 edges at (70.5, -79, 5) (-3, -79, 5) on bodies 2 in component "Topo"
fillet "Fillet2''" radius 2 5 edges at (70.5, -17.75, 7) (69.0355, 8.5355, 7) (35.25, 10, 7) (1.4645, 8.5355, 7) (0, -30, 7) on bodies 3 in component "Trinco"
fillet "Fillet7" radius 2 5 edges at (70.5, -51.75, 10) (69.0355, -77.5355, 10) (33.75, -79, 10) (-1.5355, -77.5355, 10) (-3, -37.5, 10) on bodies 2 in component "Topo"
fillet "Fillet8" radius 2 3 edges at (23.75, -1, 10) (-2.4142, -1, 9.4142) (-3, -1, 4) on bodies 2 in component "Topo"
extrude "Extrude1'" cut 1 faces at (63.1667, -40.5, 2.3333) along direction (0, 1, 0) blind 0.5 on bodies 3 bodies 3 in component "Trinco"
extrude "Extrude13" cut 1 faces at (63.5, -29.5, 3.3333) along direction (0, -1, 0) blind 0.5 on bodies 2 bodies 2 in component "Topo"
extrude "Extrude14" cut 1 faces at (31.6667, -54, 5.3333) along direction (0, -1, 0) blind 1 on bodies 2 bodies 2 in component "Topo"
fillet "Fillet3'" radius 5 1 edges at (50.5, -52.5, 0) on bodies 3 in component "Trinco"
extrude "Extrude15" add 1 faces at (-1, -19, 5.3333) along direction (1, 0, 0) blind 0.75 on bodies 2 bodies 2 in component "Topo"
extrude "Extrude16" add 1 faces at (51.5, -31.5, 2.6667) along direction (-1, 0, 0) blind 0.75 on bodies 2 bodies 2 in component "Topo"
sketch "Sketch7" plane through (0, 0, 10) normal (0, 0, 1) x (-1, 0, 0)
  line L0 (-48.5, 40) -> (-48.5, 13)
  line L1 (-48.5, 13) -> (1, 13)
  line L2 (1, 13) -> (1, 84)
  arc A0 (1, 84) -> (-2, 87) centre (-2, 84) ccw
  line L3 (-2, 87) -> (-65.5, 87)
  arc A1 (-65.5, 87) -> (-68.5, 84) centre (-65.5, 84) ccw
  line L4 (-68.5, 84) -> (-68.5, 40)
  line L5 (-68.5, 40) -> (-48.5, 40)
  line L6 (-51.5, 44.5) -> (-57.5, 44.5)
  line L7 (-57.5, 44.5) -> (-57.5, 84)
  line L8 (-57.5, 84) -> (-50.5, 84)
  line L9 (-50.5, 84) -> (-50.5, 64)
  line L10 (-50.5, 64) -> (-51.5, 62.775)
  line L11 (-51.5, 62.775) -> (-51.5, 44.5)
  line L12 (-5, 76) -> (-5, 69)
  line L13 (-5, 69) -> (-43.5, 69)
  line L14 (-43.5, 69) -> (-43.5, 76)
  line L15 (-43.5, 76) -> (-5, 76)
  line L16 (-67.5, 84) -> (-58.5, 84)
  line L17 (-58.5, 84) -> (-58.5, 44.5)
  line L18 (-58.5, 44.5) -> (-67.5, 44.5)
  line L19 (-67.5, 44.5) -> (-67.5, 84)
  line L20 (-5, 86) -> (-5, 77)
  line L21 (-5, 77) -> (-43.5, 77)
  line L22 (-43.5, 77) -> (-43.5, 86)
  line L23 (-43.5, 86) -> (-5, 86)
  line L24 (-70.5, 35.5) -> (-50.5, 35.5)
  line L25 (-50.5, 35.5) -> (-48.5, 35.5)
  line L26 (-48.5, 35.5) -> (-52.373, 40.2445)
  dimension "d131" = 140.774
  dimension "d132" = 140.774
  constraint coincident L24.end L25.start
  constraint coincident L0 L25.end
  constraint perpendicular L0 L25
  measures "d131" angle of L9 L10
  measures "d132" angle of L0 L26
extrude "Extrude17" add sketch "Sketch7" against normal up to surface (2 mm away) contours L0 L5 L26 sketch seen with x (1, 0, 0) y (0, 1, 0) z (0, 0, 1) at (0, 10, 0) bodies 2 in component "Topo"
component "Topo" placed x (1, 0, 0) y (0, 1, 0) z (0, 0, 1) at (0, -10, 0)
component "Trinco" placed x (1, 0, 0) y (0, 1, 0) z (0, 0, 1) at (0, 0, 0)
equation "d1 = 38.5 mm + 2 mm + 10 mm"
equation "d34 = d33"
equation "d52 = d53"
equation "d132 = d131"
